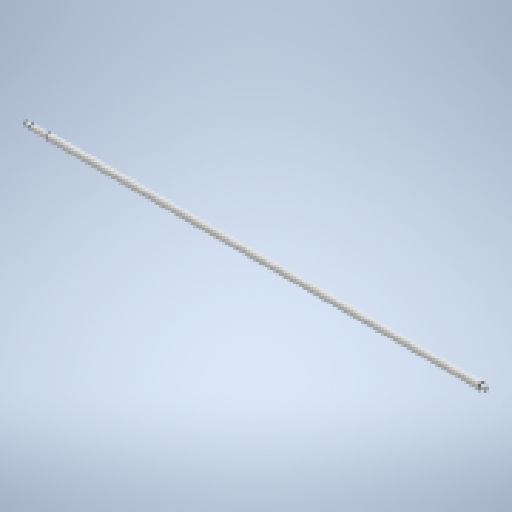
# Autodesk Inventor part: SFU1605
Saved by Autodesk Inventor 2023 (Build 270158000, 158)
## iProperties
Created: 2022-05-01
Part Number: SFU1605
Material: Generic
Document SubType Name: Modeling
Designer: plebbb
Density: 1 g/cm^3
Appearance: Default
Author: plebbb
Autodesk Inventor part; units mm, degrees
ref_plane "YZ Plane" through (0, 0, 0) normal (1, 0, 0) x (0, 1, 0)
ref_plane "XZ Plane" through (0, 0, 0) normal (0, 1, 0) x (-1, 0, 0)
ref_plane "XY Plane" through (0, 0, 0) normal (0, 0, 1) x (1, 0, 0)
sketch "Sketch1" plane through (0, 0, 0) normal (0, 0, 1) x (1, 0, 0)
  line L0 (0, 0) -> (0, 5)
  line L1 (0, 5) -> (15, 5)
  line L2 (15, 5) -> (15, 6)
  line L3 (15, 6) -> (54, 6)
  line L4 (54, 6) -> (54, 8)
  line L5 (54, 8) -> (1089, 8)
  line L6 (1089, 8) -> (1089, 5)
  line L7 (1089, 5) -> (1100, 5)
  line L8 (1100, 5) -> (1100, 0)
  line L9 (1100, 0) -> (0, 0)
  line L10 (0, 0) -> (1100, 0)
  dimension "d0" = 5
  dimension "d1" = 6
  dimension "d2" = 8
  dimension "d3" = 5
  dimension "d4" = 11
  dimension "d6" = 39
  dimension "d8" = 15
  dimension "d9" = 1100
  constraints: 23 end point, 8 perpendicular, 2 vertical, 1 collinear
  measures "d0" distance of L0.start L0.end
  measures "d1" distance from line of L0.start L3
  measures "d2" distance from line of L0.start L5
  measures "d3" distance from line of L0.start L7
  measures "d4" distance of L6.end L7.end
  measures "d6" distance of L3.end L2.end
  measures "d8" distance of L0.end L1.end
  measures "d9" distance between parallel lines of L0 L8
revolve "Revolution1" add sketch "Sketch1" angle 360 about axis through (0, 0, 0) along (1, 0, 0)
body "Solid1"
